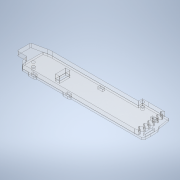
# Autodesk Inventor part: Laser-Slot-Side
Saved by Autodesk Inventor 2021 (Build 250183000, 183)
## iProperties
Created: 2020-06-23
Part Number: Laser-Slot-Side
Material: Acrylic, Clear
Document SubType Name: Modeling
Designer: lucas
Density: 1.19 g/cm^3
Appearance: Transparent - Clear
Project: 4Wire-Laser
Author: lucas
Revision Number: RLS_001
Autodesk Inventor part; units mm, degrees
ref_plane "YZ Plane" through (0, 0, 0) normal (1, 0, 0) x (0, 1, 0)
ref_plane "XZ Plane" through (0, 0, 0) normal (0, 1, 0) x (-1, 0, 0)
sketch "Sketch1" plane through (0, 0, 0) normal (0, 1, 0) x (-1, 0, 0)
  arc A0 (-6.5171, 18.4998) -> (-6.2733, 11.0691) centre (108.3458, 18.5495) ccw
  line L0 (82.9264, 7.5998) -> (82.9264, 17.5998) construction
  line L1 (82.9264, 7.5998) -> (86.9264, 7.5998) construction
  line L2 (86.9264, 7.5998) -> (86.9264, 17.5998) construction
  line L3 (86.9264, 17.5998) -> (82.9264, 17.5998) construction
  line L4 (82.9264, 17.5998) -> (82.9264, 7.5998) construction
  line L5 (115.5711, 18.5384) -> (115.5711, 1.6532)
  line L6 (-6.5171, 23.2498) -> (-6.5171, 18.4998)
  line L7 (3.4264, 1.5998) -> (3.4264, 3.5998) construction
  line L8 (3.4264, 1.5998) -> (7.9264, 1.5998) construction
  line L9 (3.4264, 3.5998) -> (7.9264, 3.5998) construction
  line L10 (7.9264, 1.5998) -> (7.9264, 3.5998) construction
  line L11 (59.4264, 1.5998) -> (59.4263, 3.5871) construction
  line L12 (54.9264, 1.5998) -> (54.9264, 3.5998) construction
  line L13 (54.9264, 1.5998) -> (59.4264, 1.5998) construction
  line L14 (54.9264, 3.5998) -> (59.4263, 3.5871) construction
  line L15 (17.4264, -0.0002) -> (107.9264, -0.0002)
  line L16 (-2.0736, 20.5998) -> (-2.0736, 11.5998) construction
  line L17 (-6.5171, 22.5998) -> (113.8037, 22.5998) construction
  line L18 (-2.0736, 11.5998) -> (-4.0736, 11.5998) construction
  line L19 (-4.0736, 11.5998) -> (-4.0736, 20.5998) construction
  line L20 (-4.0736, 20.5998) -> (-2.0736, 20.5998) construction
  line L21 (-2.5736, 3.5998) -> (62.4264, 3.5998) construction
  line L22 (-2.5736, 12.5998) -> (62.4264, 12.5998) construction
  line L23 (62.4264, 12.5998) -> (92.4264, 12.5998) construction
  line L24 (107.9264, 18.4998) -> (-6.5171, 18.4998) construction
  line L25 (29.9264, 12.5998) -> (29.9264, -9.6247) construction
  line L26 (29.9264, 12.5998) -> (52.1508, 12.5998) construction
  line L27 (17.4264, -0.0002) -> (17.4264, -4.0002)
  circle A1 centre (107.9264, 18.4612) radius 1.6
  arc A2 (115.5711, 18.4612) -> (111.7578, 25.1151) centre (107.9264, 18.4998) ccw
  arc A3 (114.6882, 22.0663) -> (113.8037, 22.5998) centre (113.8037, 21.5998) ccw construction
  arc A4 (107.9264, -0.0002) -> (112.0053, 0.4551) centre (107.9264, 18.4998) ccw
  line L28 (107.9264, 18.4998) -> (112.0053, 0.4551) construction
  line L29 (107.9264, 18.4998) -> (107.9264, -0.0002) construction
  line L30 (112.0053, 0.4551) -> (115.5711, 1.2611)
  line L31 (115.5711, 1.2611) -> (115.5711, 1.6532)
  arc A5 (107.9264, -0.0002) -> (112.0053, 0.4551) centre (107.9264, 18.4998) ccw
  arc A6 (115.5711, 1.6532) -> (115.5712, 1.6532) centre (107.9264, 18.4998) ccw
  line L32 (107.9264, 18.4998) -> (10.3873, -3.5485) construction
  line L33 (107.9264, 18.4998) -> (207.9264, 18.4998) construction
  line L34 (17.4264, -4.0002) -> (23.4264, -4.0002)
  line L35 (23.4264, -4.0002) -> (23.4264, -0.0002)
  circle A7 centre (20.5552, -1.25) radius 1.6
  line L36 (86.9639, 17.6373) -> (86.9639, 7.5623)
  line L37 (86.9639, 7.5623) -> (82.8889, 7.5623)
  line L38 (82.8889, 7.5623) -> (82.8889, 17.6373)
  line L39 (82.8889, 17.6373) -> (86.9639, 17.6373)
  line L40 (59.5013, 3.6619) -> (54.8514, 3.675)
  line L41 (54.8514, 3.675) -> (54.8514, 1.5248)
  line L42 (54.8514, 1.5248) -> (59.5014, 1.5248)
  line L43 (59.5014, 1.5248) -> (59.5013, 3.6619)
  line L44 (8.0014, 3.6748) -> (3.3514, 3.6748)
  line L45 (3.3514, 3.6748) -> (3.3514, 1.5248)
  line L46 (3.3514, 1.5248) -> (8.0014, 1.5248)
  line L47 (8.0014, 1.5248) -> (8.0014, 3.6748)
  line L48 (-1.9986, 20.6748) -> (-1.9986, 11.5248)
  line L49 (-1.9986, 11.5248) -> (-4.1486, 11.5248)
  line L50 (-4.1486, 11.5248) -> (-4.1486, 20.6748)
  line L51 (-4.1486, 20.6748) -> (-1.9986, 20.6748)
  line L52 (111.2567, 25.2498) -> (75.3036, 25.2498)
  line L53 (75.3036, 25.2498) -> (-4.5171, 25.2498)
  arc A8 (111.7578, 25.1151) -> (111.2567, 25.2498) centre (111.2567, 24.2498) ccw
  arc A9 (-4.5171, 25.2498) -> (-6.5171, 23.2498) centre (-4.5171, 23.2498) ccw
  line L54 (3.4264, 1.5998) -> (-13.0902, 1.5998) construction
  line L55 (3.4264, 1.5998) -> (19.9429, 1.5998) construction
  line L56 (17.4264, -4.0002) -> (-2.4009, -4.0002)
  line L57 (17.4264, -4.0002) -> (40.1404, -4.0002) construction
  arc A10 (-6.2733, 11.0691) -> (-4.7912, 8.3543) centre (-2.0736, 11.5998) ccw
  arc A11 (-4.0856, 7.0247) -> (-2.4009, -4.0002) centre (107.9264, 18.4998) ccw
  arc A12 (-4.0856, 7.0247) -> (-4.7912, 8.3543) centre (-6.0752, 6.8208) ccw
  point P0 (-6.4023, 13.4157)
  point P1 (114.3787, 22.5998)
  point P2 (111.5153, 25.2498)
  point P3 (-1.5232, 1.5998)
  point P4 (-4.7755, 7.5623)
  dimension "d11" = 4
  dimension "d12" = 10
  dimension "d36" = 110
  dimension "d37" = 18.5
  dimension "d38" = 25
  dimension "d39" = 22.6
  dimension "d40" = 2
  dimension "d41" = 9
  dimension "d42" = 2
  dimension "d43" = 1.6
  dimension "d44" = 2
  dimension "d45" = 4.5
  dimension "d47" = 65
  dimension "d48" = 9
  dimension "d50" = 10
  dimension "d51" = 3.6
  dimension "d52" = 7.6
  dimension "d53" = 5
  dimension "d54" = 1.6
  dimension "d58" = 4.5
  dimension "d59" = 2
  dimension "d60" = 90.5
  dimension "d61" = 4
  dimension "d64" = 3.2
  dimension "d65" = 1
  dimension "d77" = 11.8
  dimension "d81" = 12.737
  dimension "d82" = 100
  dimension "d83" = 167.263
  dimension "d85" = 6
  dimension "d86" = 3.2
  dimension "d87" = 0.0375
  dimension "d88" = 0.075
  dimension "d89" = 0.075
  dimension "d90" = 0.075
  dimension "d92" = 57
  dimension "d93" = 47
  dimension "d94" = 6.75
  dimension "d95" = 1
  dimension "d96" = 2
  dimension "d134" = 180
  dimension "d137" = 180
  dimension "d139" = 8
  dimension "d157" = 2
  constraints: 116 end point, 28 point on circle, 13 centre point, 12 horizontal, 10 perpendicular, 10 tangent, 7 point on line, 6 parallel, 5 equal length, 5 vertical, 4 coincident, 1 midpoint, 13 other
  measures "d11" distance of L0.end L2.end
  measures "d12" distance of L2.end L1.end
  measures "d36" distance from line of L16 L24.start
  measures "d37" distance from line of L15 L24.start
  measures "d38" distance from line of L0 L24.start
  measures "d39" distance between parallel lines of L15 L17
  measures "d40" distance from line of L17 L16.start
  measures "d41" distance of L16.start L16.end
  measures "d42" distance of L16.end L18.end
  measures "d43" distance between parallel lines of L13 L15
  measures "d44" distance of L12.start L12.end
  measures "d45" distance of L12.end L11.end
  measures "d47" distance of L21.start L21.end
  measures "d48" distance between parallel lines of L21 L22
  measures "d50" diameter of L3 L23
  measures "d51" distance between parallel lines of L15 L21
  measures "d52" distance between parallel lines of L15 L1
  measures "d53" distance between parallel lines of L17 L3
  measures "d54" distance between parallel lines of L15 L8
  measures "d58" distance of L7.end L9.end
  measures "d59" distance of L7.start L7.end
  measures "d60" horizontal distance of L15.start L24.start
  measures "d61" distance of L15.start L27.end
  measures "d64" diameter of A1
  measures "d65" radius of A3
  measures "d77" diameter of L24.start L23
  measures "d81" angle of L29 L28
  measures "d82" distance of L28.start L32.end
  measures "d83" angle of L32 L33
  measures "d85" distance of L27.end L34.end
  measures "d86" diameter of A7
  measures "d87" distance between parallel lines of L2 L36
  measures "d88" distance between parallel lines of L11 L43
  measures "d89" distance between parallel lines of L10 L47
  measures "d90" distance between parallel lines of L20 L51
  measures "d92" distance between parallel lines of L12 L16
  measures "d93" distance between parallel lines of L10 L12
  measures "d94" distance from line of L52 A5.centre
  measures "d95" radius of A8
  measures "d96" radius of A9
  measures "d134" angle of L54 L55
  measures "d137" angle of L56 L57
  measures "d139" distance between parallel lines of L21 L18
  measures "d157" radius of A12
extrude "Extrusion1" add sketch "Sketch1" along normal blind 2 contours L6 A9 L53 L52 A6 L15 A7 L27 L56 A11 A12 A10 A0 | L52 A8 A2 L5 A6 A4 | L27 L15 A7 L35 L34 | L31 L30 A6
sketch "Sketch3" plane through (0, 2, 0) normal (0, 1, 0) x (1, 0, 0)
  arc A0 (-1.8315, -21.7932) -> (-1.8017, -20.6277) centre (-107.9198, -18.4998) ccw
  arc A1 (-1.8017, -20.6277) -> (1.5761, -19.4924) centre (-7.1257, 0.8052) ccw
  arc A2 (1.5761, -19.4924) -> (1.5804, -18.2896) centre (-107.9198, -18.4998) ccw
  arc A3 (1.5804, -18.2896) -> (-1.7892, -17.1302) centre (-7.2662, -38.5246) ccw
  arc A4 (-1.7892, -17.1302) -> (-1.8106, -15.9645) centre (-107.9198, -18.4998) ccw
  arc A5 (-1.8106, -15.9645) -> (1.5141, -14.6819) centre (-8.0709, 5.2139) ccw
  arc A6 (1.5141, -14.6819) -> (1.4655, -13.4801) centre (-107.9198, -18.4998) ccw
  arc A7 (1.4655, -13.4801) -> (-1.9518, -12.4698) centre (-6.4838, -34.0841) ccw
  arc A8 (-1.9518, -12.4698) -> (-2.0244, -11.3062) centre (-107.9198, -18.4998) ccw
  arc A9 (-2.0244, -11.3062) -> (1.2408, -9.8788) centre (-9.2089, 9.5768) ccw
  arc A10 (1.2408, -9.8788) -> (1.1395, -8.6803) centre (-107.9198, -18.4998) ccw
  arc A11 (1.1395, -8.6803) -> (-2.3189, -7.8211) centre (-5.8971, -29.6136) ccw
  arc A12 (-2.3189, -7.8211) -> (-2.4426, -6.6618) centre (-107.9198, -18.4998) ccw
  arc A13 (-2.4426, -6.6618) -> (0.7567, -5.0924) centre (-10.5374, 13.8855) ccw
  arc A14 (0.7567, -5.0924) -> (0.6029, -3.8994) centre (-107.9198, -18.4998) ccw
  arc A15 (0.6029, -3.8994) -> (-2.8899, -3.193) centre (-5.5074, -25.1216) ccw
  arc A16 (-3.0644, -2.0402) -> (0.0629, -0.3318) centre (-12.0539, 18.1317) ccw
  arc A17 (-2.8899, -3.193) -> (-3.0644, -2.0402) centre (-107.9198, -18.4998) ccw
  arc A18 (0.0629, -0.3318) -> (-0.1432, 0.8533) centre (-107.9198, -18.4998) ccw
  arc A19 (-0.1432, 0.8533) -> (-3.6636, 1.4056) centre (-5.3154, -20.6168) ccw
  arc A20 (-3.8859, 2.5451) -> (-1.3941, 4) centre (-13.7518, 22.3031) ccw
  arc A21 (-3.661, 1.4011) -> (-3.8859, 2.5451) centre (-107.9181, -18.4995) ccw
  arc A22 (-1.0944, 5.564) -> (-1.0963, 5.5643) centre (-5.3197, -16.1124) ccw
  line L0 (0.5131, 4) -> (-17.4264, 4.0002)
  line L1 (-17.4264, 4.0002) -> (-17.4264, 0.0002)
  line L2 (-17.4264, 0.0002) -> (-107.9264, 0.0002)
  arc A23 (-107.9264, 0.0002) -> (-112.0053, -0.4551) centre (-107.9264, -18.4998) ccw
  line L3 (-115.5711, -16.7442) -> (-115.5711, -18.5384)
  arc A24 (-115.5711, -18.5384) -> (-114.6882, -22.0663) centre (-107.9264, -18.4998) ccw
  arc A25 (-114.6882, -22.0663) -> (-113.8037, -22.5998) centre (-113.8037, -21.5998) ccw construction
  line L4 (-113.8037, -22.5998) -> (6.5171, -22.5998) construction
  line L5 (6.5171, -22.5998) -> (6.5171, -18.4998)
  arc A26 (6.5171, -18.4998) -> (6.4023, -13.4156) centre (-108.3467, -18.5494) ccw
  arc A27 (6.4023, -13.4156) -> (5.0884, -11.6257) centre (4.4043, -13.505) ccw
  line L6 (5.0884, -11.6257) -> (3.7578, -11.1414)
  arc A28 (2.4503, -9.4258) -> (3.7578, -11.1414) centre (4.4437, -9.2626) ccw
  arc A29 (2.4503, -9.4258) -> (0.5131, 4) centre (-107.9264, -18.4998) ccw
  line L7 (-112.0558, -0.4665) -> (-124.7005, -3.3248)
  line L8 (-125.48, -4.2973) -> (-125.5125, -15.7414)
  arc A30 (-124.7005, -3.3248) -> (-125.48, -4.2973) centre (-124.48, -4.3001) ccw
  arc A31 (-125.5125, -15.7414) -> (-124.5153, -16.7442) centre (-124.5125, -15.7442) ccw
  arc A32 (-107.9264, 0.0002) -> (-112.0053, -0.4551) centre (-107.9264, -18.4998) ccw
  line L9 (-112.0053, -0.4551) -> (-124.7005, -3.3248)
  circle A33 centre (-107.9264, -18.4612) radius 1.6
  line L10 (-124.5153, -16.7442) -> (-115.5711, -16.7442)
  line L11 (-115.5711, -1.2611) -> (-115.5711, -18.4612) projected
  line L12 (-84.4264, -17.5998) -> (-84.4264, -7.5998)
  line L13 (-80.4264, -17.5998) -> (-84.4264, -17.5998)
  line L14 (-80.4264, -7.5998) -> (-80.4264, -17.5998)
  line L15 (-80.4264, -7.5998) -> (-84.4264, -7.5998)
  line L16 (2.4009, 4.0002) -> (-23.4264, 4.0002) projected
  line L17 (-23.4264, 4.0002) -> (-23.4264, 0.0002) projected
  circle A34 centre (-20.5552, 1.25) radius 1.6 projected
  line L18 (-86.9639, -17.6373) -> (-86.9639, -7.5623) projected
  line L19 (-82.8889, -17.6373) -> (-86.9639, -17.6373) projected
  line L20 (-82.8889, -7.5623) -> (-82.8889, -17.6373) projected
  line L21 (-86.9639, -7.5623) -> (-82.8889, -7.5623) projected
  arc A35 (4.5171, -25.2498) -> (6.5171, -23.2498) centre (4.5171, -23.2498) ccw projected
  line L22 (6.5171, -23.2498) -> (6.5171, -18.4998) projected
  line L23 (-111.2567, -25.2498) -> (4.5171, -25.2498) projected
  arc A36 (-115.5711, -18.4612) -> (-111.7578, -25.1151) centre (-107.9264, -18.4998) ccw projected
  arc A37 (-111.7578, -25.1151) -> (-111.2567, -25.2498) centre (-111.2567, -24.2498) ccw projected
  arc A38 (-1.8183, -25.2498) -> (1.4268, -24.301) centre (-6.375, -3.6407) ccw
  arc A39 (1.4268, -24.301) -> (1.484, -23.0995) centre (-107.9198, -18.4997) ccw
  arc A40 (1.484, -23.0995) -> (-1.8315, -21.7932) centre (-8.2429, -42.9264) ccw
  point P0 (-115.5711, -1.6532)
  point P1 (-3.6618, 1.4055)
  point P2 (-21.5541, 0.0002)
  point P3 (-19.5562, 0.0002)
  dimension "d79" = 167.263
  dimension "d97" = 2.518
  constraints: 74 point on circle, 37 centre point, 30 end point, 2 point on line, 2 tangent, 1 collinear, 1 perpendicular
  measures "d79" angle of L2 L7
extrude "Extrusion2" add sketch "Sketch3" along normal blind 4 contours A40 A39 A38 L23 A22 A34 L2 L1 L0 A20 A21 A19 A18 A16 A17 A15 A14 A13 A12 A11 A10 A9 A8 A7 A6 A5 A4 A3 A2 A1 A0 | L23 A37 A36 A24 L3 L11 L7 L9 A23 L2 A34 A22 | L2 L17 L16 L1 A22 A34 | A34 A22 L1 L2 | A22 L1 L0 | L10 A31 L8 A30 L7 L11 | L20 L15 L14 L13
ref_plane "Work Plane1" through (0, 2, 0) normal (0, 1, 0) x (1, 0, 0)
split body "Split1" result two bodies by plane through (0, 2, 0) normal (0, 1, 0) first body at (-36.0445, 5.5, 14.2956)
fillet "Fillet1" radius 0.25 5 edges at (-23.4264, 4, -4.0002) (-23.4264, 4, -0.0002) (-115.5711, 4, 16.7442) (-23.4264, 1, -4.0002) (-23.4264, 1, -0.0002)
sketch "Sketch5" plane through (0, 6, 0) normal (0, 1, 0) x (1, 0, 0)
  line L0 (-82.8889, -7.5623) -> (-82.8889, -17.6373) projected
  line L1 (-86.9639, -7.5623) -> (-86.9639, -17.6373) projected
  point P0 (0, 0)
  point P1 (-80.3514, -17.6748)
  constraints: 1 coincident
hole "Hole2" at (-82.8889, 6, 17.6373) at (-86.9639, 6, 17.6373) at (-86.9639, 6, 7.5623) at (-82.8889, 6, 7.5623) direction (0, -1, 0) diameter 0.3 end through all bodies 2
sketch "Sketch6" plane through (0, 0, 0) normal (0, -1, 0) x (1, 0, 0)
  arc A0 (-82.8889, 17.4873) -> (-83.0389, 17.6373) centre (-82.8889, 17.6373) ccw projected
  line L0 (-86.9639, 17.6373) -> (-86.9639, 7.5623) projected
  point P0 (0, 0)
  point P1 (-82.8889, 7.5248)
  constraints: 2 coincident
hole "Hole3" at (-82.8889, 0, 17.6373) at (-86.9639, 0, 17.6373) at (-86.9639, 0, 7.5623) at (-82.8889, 0, 7.5248) direction (0, 1, 0) diameter 0.3 end through all bodies 3
fillet "Fillet2" radius 0.25 1 edges at (-115.5711, 1, 1.2611)
sketch "Sketch7" plane through (0, 0, 0) normal (0, -1, 0) x (1, 0, 0)
  line L0 (-83.0389, 17.6373) -> (-86.8139, 17.6373) construction
  line L1 (-86.8139, 17.6373) -> (-83.0389, 17.6373) projected
  line L2 (-84.9264, 17.6373) -> (-84.9264, 25.2498) construction
  line L3 (-84.9264, 25.2498) -> (-69.9264, 25.2498) construction
  line L4 (-84.9264, 25.2498) -> (-67.9264, 25.2498) construction
  line L5 (-111.2567, 25.2498) -> (-1.8183, 25.2498) projected
  line L6 (-84.9264, 25.2498) -> (-101.9264, 25.2498) construction
  line L7 (-101.9264, 25.2498) -> (-101.9264, 23.6498) construction
  line L8 (-67.9264, 25.2498) -> (-67.9264, 23.6498) construction
  line L9 (-103.9264, 24.6498) -> (-99.9264, 24.6498)
  line L10 (-99.9264, 24.6498) -> (-99.9264, 22.6498)
  line L11 (-99.9264, 22.6498) -> (-103.9264, 22.6498)
  line L12 (-103.9264, 22.6498) -> (-103.9264, 24.6498)
  line L13 (-103.9264, 24.6498) -> (-99.9264, 22.6498) construction
  line L14 (-99.9264, 24.6498) -> (-103.9264, 22.6498) construction
  line L15 (-69.9264, 24.6498) -> (-65.9264, 24.6498)
  line L16 (-65.9264, 24.6498) -> (-65.9264, 22.6498)
  line L17 (-65.9264, 22.6498) -> (-69.9264, 22.6498)
  line L18 (-69.9264, 22.6498) -> (-69.9264, 24.6498)
  line L19 (-69.9264, 24.6498) -> (-65.9264, 22.6498) construction
  line L20 (-65.9264, 24.6498) -> (-69.9264, 22.6498) construction
  arc A0 (-103.9264, 26.6498) -> (-105.8342, 25.2498) centre (-103.9264, 24.6498) ccw
  arc A1 (-98.0185, 25.2498) -> (-99.9264, 26.6498) centre (-99.9264, 24.6498) ccw
  arc A2 (-69.9264, 26.6498) -> (-71.8342, 25.2498) centre (-69.9264, 24.6498) ccw
  arc A3 (-64.0185, 25.2498) -> (-65.9264, 26.6498) centre (-65.9264, 24.6498) ccw
  line L21 (-69.9264, 26.6498) -> (-65.9264, 26.6498)
  line L22 (-103.9264, 26.6498) -> (-99.9264, 26.6498)
  line L23 (-98.0185, 25.2498) -> (-105.8342, 25.2498)
  line L24 (-64.0185, 25.2498) -> (-71.8342, 25.2498)
  point P0 (0, 0)
  dimension "d142" = 17
  dimension "d144" = 17
  dimension "d145" = 1.6
  dimension "d146" = 1.6
  dimension "d147" = 4
  dimension "d148" = 2
  dimension "d149" = 4
  dimension "d150" = 2
  dimension "d151" = 2
  dimension "d152" = 2
  dimension "d153" = 2
  dimension "d154" = 2
  constraints: 44 end point, 8 point on circle, 5 midpoint, 4 centre point, 4 horizontal, 4 parallel, 3 coincident, 3 vertical, 2 collinear, 2 perpendicular, 2 point on line, 5 other
  measures "d142" distance of L2.end L4.end
  measures "d144" distance of L2.end L6.end
  measures "d145" distance of L6.end L7.end
  measures "d146" distance of L4.end L8.end
  measures "d147" distance of L10.end L11.end
  measures "d148" distance of L9.end L10.end
  measures "d149" distance of L16.end L17.end
  measures "d150" distance of L15.end L16.end
  measures "d151" radius of A0
  measures "d152" radius of A1
  measures "d153" radius of A2
  measures "d154" radius of A3
extrude "Extrusion3" cut sketch "Sketch7" against normal blind 2 contours L9 L10 L11 L12 | L15 L16 L17 L18 bodies 3
extrude "Extrusion5" add sketch "Sketch7" against normal blind 2 contours A0 L22 A1 L5 | A2 L21 A3 L5 bodies 3
fillet "Fillet4" radius 0.15 26 edges at (-1.8183, 4, 25.2498) (-3.8859, 4, -2.5451) (-3.6618, 4, -1.4055) (-3.0644, 4, 2.0402) (-2.8899, 4, 3.193) (-2.4426, 4, 6.6618) (-2.3189, 4, 7.8211) (-2.0244, 4, 11.3062) (-1.9518, 4, 12.4698) (-1.8106, 4, 15.9645) (-1.7892, 4, 17.1302) (-1.8017, 4, 20.6277) (-1.8315, 4, 21.7932) (1.4268, 4, 24.301) (1.484, 4, 23.0995) (1.5761, 4, 19.4924) (1.5804, 4, 18.2896) (1.5141, 4, 14.6819) (1.4655, 4, 13.4801) (1.2408, 4, 9.8788) (1.1395, 4, 8.6803) (0.7567, 4, 5.0924) (0.6029, 4, 3.8994) (0.0629, 4, 0.3318) (-0.1432, 4, -0.8533) (2.4009, 1, -4.0002)
fillet "Fillet5" radius 0.4 4 edges at (-98.0185, 1, 25.2498) (-105.8342, 1, 25.2498) (-71.8342, 1, 25.2498) (-64.0185, 1, 25.2498)
